V3D Leadscrew Alignment Jig v17 (Autodesk Fusion 360 design; units mm, degrees)
Autodesk Fusion 360 part; units mm, degrees
sketch "Sketch1" plane through (0, 0, 0) normal (0, 0, 1) x (1, 0, 0)
  line L0 (0, 0) -> (0, 8.85)
  line L1 (0, 8.85) -> (9, 8.85)
  line L2 (9, 8.85) -> (9, 21.15)
  line L3 (9, 21.15) -> (0, 21.15)
  line L4 (0, 21.15) -> (0, 30)
  line L5 (0, 0) -> (12, 0)
  line L6 (26, 30) -> (31.5, 35.5)
  line L7 (31.5, 35.5) -> (31.5, 63.5)
  line L8 (0, 30) -> (12, 30)
  line L9 (21.5, 47.35) -> (21.5, 55.65) construction
  line L10 (17, 63.5) -> (31.5, 63.5)
  arc A0 (21.5, 47.35) -> (21.5, 55.65) centre (21.5, 51.5) ccw
  line L11 (21.5, 47.35) -> (17, 47.35)
  line L12 (17, 47.35) -> (12, 30)
  line L13 (21.5, 55.65) -> (17, 55.65)
  line L14 (17, 55.65) -> (17, 63.5)
  line L15 (30, -8.65) -> (30, -0.35) construction
  line L16 (30, -0.35) -> (25.5, -0.35)
  line L17 (30, -8.65) -> (25.5, -8.65)
  arc A1 (30, -8.65) -> (30, -0.35) centre (30, -4.5) ccw
  line L18 (12, 0) -> (25.5, -0.35)
  line L19 (25.5, -8.65) -> (25.5, -16.5)
  line L20 (25.5, -16.5) -> (40, -16.5)
  line L21 (40, -16.5) -> (40, 7.5)
  line L22 (40, 7.5) -> (26, 7.5)
  line L23 (26, 7.5) -> (26, 30)
  dimension "d3" = 9
  dimension "d4" = 12.3
  dimension "d6" = 30
  dimension "d7" = 21.5
  dimension "d8" = 51.5
  dimension "d10" = 8.3
  dimension "d13" = 17
  dimension "d14" = 10
  dimension "d15" = 12
  dimension "d20" = 12
  dimension "d22" = 12
  dimension "d25" = 4.5
  dimension "d26" = 30
  dimension "d27" = 12
  dimension "d28" = 10
  dimension "d29" = 12
  dimension "d32" = 26
  dimension "d33" = 45
  constraint perpendicular L0 L1
  constraint perpendicular L0 L3
  constraint perpendicular L3 L4
  constraint perpendicular L5 L7
  constraint collinear L0 L4
  constraint perpendicular L0 L5
  constraint coincident L0.start L5.start
  constraint horizontal L5
  constraint perpendicular L4 L8
  constraint equal L0 L4
  constraint coincident A0.centre L9
  constraint vertical L9
  constraint coincident L7 L10.end
  constraint tangent A0 L11
  constraint tangent A0 L13
  constraint perpendicular L13 L14
  constraint coincident L11.end L14
  constraint horizontal L10
  constraint equal A0 A1
  constraint vertical L15
  constraint tangent L16 A1
  constraint tangent L17 A1
  constraint equal L13 L16
  constraint equal L16 L17
  constraint perpendicular L17 L19
  constraint perpendicular L19 L20
  constraint perpendicular L17 L21
  constraint horizontal L16
  constraint perpendicular L22 L23
  constraint horizontal L22
  constraint coincident L8 L6.start
  measures "d3" distance of L2 L4
  measures "d4" distance of L1 L3
  measures "d6" distance of L5 L8
  measures "d7" distance of L0 A0.centre
  measures "d8" distance of L5 A0.centre
  measures "d10" diameter of A0
  measures "d13" distance of L4 L14
  measures "d14" distance of L7 A0.centre
  measures "d15" distance of A0.centre L10
  measures "d20" distance of L0.start L5.end
  measures "d22" distance of L0 L8.end
  measures "d25" distance of L5 A1.centre
  measures "d26" distance of L0 A1.centre
  measures "d27" distance of A1.centre L20
  measures "d28" distance of A1.centre L21
  measures "d29" vertical distance of A1.centre L21.end
  measures "d32" distance of L0 L23
  measures "d33" angle of L6 L23
extrude "Extrude1" add sketch "Sketch1" along normal blind 18
chamfer "Chamfer1" distance 2 distance2 3 13 edges at (31.5, 49.5, 18) (28.75, 32.75, 18) (28.75, 32.75, 0) (17, 63.5, 9) (14.5, 38.675, 18) (14.5, 38.675, 0) (17, 59.575, 18) (17, 59.575, 0) (33, 7.5, 18) (40, -4.5, 18) (33, 7.5, 0) (25.5, -12.575, 18) (25.5, -12.575, 0) measured on face at (20.3333, 19.55, 18) measured on face at (20.3333, 19.55, 18) measured on face at (27.8333, 31.8333, 6) measured on face at (21.8333, 63.5, 6) measured on face at (20.3333, 19.55, 18) measured on face at (15.3333, 41.5667, 6) measured on face at (20.3333, 19.55, 18) measured on face at (20.3333, 19.55, 0) measured on face at (20.3333, 19.55, 18) measured on face at (20.3333, 19.55, 18) measured on face at (35.3333, 7.5, 12) measured on face at (20.3333, 19.55, 18) measured on face at (25.5, -13.8833, 12)
chamfer "Chamfer2" distance 4 angle 45 3 edges at (31.5, 63.5, 7.5) (40, -16.5, 7.5) (40, 7.5, 8.5)
chamfer "Chamfer3" distance 2 angle 45 3 edges at (17, 55.65, 9) (17, 47.35, 8.5) (25.5, -8.65, 8.5)
chamfer "Chamfer4" distance 1.5 angle 45 4 edges at (0, 21.15, 9) (0, 8.85, 9) (0, 30, 9) (0, 0, 9)
chamfer "Chamfer5" distance 2 angle 45 4 edges at (5.25, 21.15, 18) (5.25, 8.85, 18) (5.25, 21.15, 0) (5.25, 8.85, 0)
chamfer "Chamfer7" distance 1 angle 45 12 edges at (25.65, 51.5, 0) (20.25, 55.65, 0) (20.811, 47.35, 0) (25.65, 51.5, 18) (20.2907, 47.35, 18) (20.25, 55.65, 18) (34.15, -4.5, 18) (28.75, -8.65, 18) (27.75, -0.35, 18) (34.15, -4.5, 0) (27.75, -0.35, 0) (29.25, -8.65, 0)
